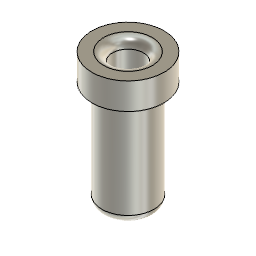
按钮头 (Autodesk Fusion 360 design; units mm, degrees)
part number: 2025-10-23-14-32-01-350
Autodesk Fusion 360 part; units mm, degrees
sketch "Sketch1" plane through (0, 0, 0) normal (0, 0, 1) x (1, 0, 0)
  circle A0 centre (0, 0) radius 2.95
  dimension "d1" = 5.9
  constraint coincident A0.centre origin
  measures "d1" diameter of A0
extrude "Extrude1" add sketch "Sketch1" along normal blind 12
sketch "Sketch2" plane through (0, 0, 12) normal (0, 0, 1) x (-1, 0, 0)
  circle A0 centre (0, 0) radius 2.95
  circle A1 centre (0, 0) radius 4.084
  constraint coincident A0.centre A1.centre
extrude "Extrude2" add sketch "Sketch2" along normal blind 3 contours A0 | A1
sketch "Sketch3" plane through (0, 0, 15) normal (0, 0, 1) x (-1, 0, 0)
  circle A0 centre (0, 0) radius 4.084
  circle A1 centre (0, 0) radius 1.75
  dimension "d6" = 3.5
  constraint concentric A0 A1
  measures "d6" diameter of A1
extrude "Extrude3" cut sketch "Sketch3" against normal blind 4 contours A1
fillet "Fillet1" radius 1 1 edges at (-2.7504, -1.0668, 0)
fillet "Fillet2" radius 1 1 edges at (1.6316, -0.6328, 15)
